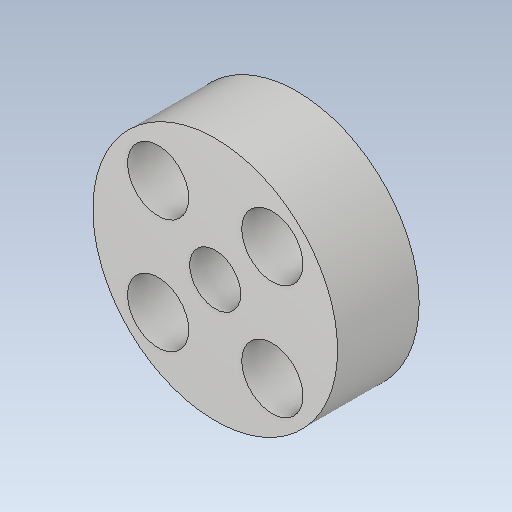
# Autodesk Inventor part: 新型３脚最終段カム
Saved by Autodesk Inventor 2020 (Build 240168000, 168)
## iProperties
Created: 2019-04-17
Part Number: 新型３脚最終段カム
Material: アルミニウム 2014-T4
Document SubType Name: Modeling
Designer: tanjihayato
Density: 2.8 g/cm^3
Appearance: サテン
Mass: 0.89504 g
Surface Area: 4.92837 cm^2
Volume: 0.319657 cm^3
Author: tanjihayato
Autodesk Inventor part; units mm, degrees
ref_plane "YZ Plane" through (0, 0, 0) normal (1, 0, 0) x (0, 1, 0)
ref_plane "XZ Plane" through (0, 0, 0) normal (0, 1, 0) x (-1, 0, 0)
ref_plane "XY Plane" through (0, 0, 0) normal (0, 0, 1) x (1, 0, 0)
sketch "スケッチ1" plane through (0, 0, 0) normal (0, 0, 1) x (1, 0, 0)
  circle A0 centre (0, 0) radius 8
  circle A1 centre (0, 0) radius 6
  circle A2 centre (0, 0) radius 1.25
  circle A3 centre (-2.8, -2.8) radius 1.5
  circle A4 centre (-2.8, 2.8) radius 1.5
  circle A5 centre (2.8, 2.8) radius 1.5
  circle A6 centre (2.8, -2.8) radius 1.5
  circle A7 centre (0, 0) radius 6
  dimension "d0" = 16
  dimension "d1" = 12
  constraints: 8 centre point, 2 coincident, 5 other
  measures "d0" diameter of A0
  measures "d1" diameter of A1
extrude "押し出し1" add sketch "スケッチ1" along normal blind 4 contours A1
